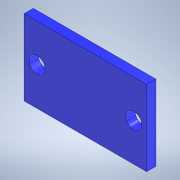
# Autodesk Inventor part: LogicLevelConverter
Saved by Autodesk Inventor 2021.2 (Build 252289000, 289)
## iProperties
Created: 2021-09-30
Part Number: LogicLevelConverter
Material: PET Plastic
Document SubType Name: Modeling
Designer: Roger
Density: 1.541 g/cm^3
Appearance: Blue - Wall Paint - Glossy
Author: Roger
Autodesk Inventor part; units mm, degrees
ref_plane "YZ Plane" through (0, 0, 0) normal (1, 0, 0) x (0, 1, 0)
ref_plane "XZ Plane" through (0, 0, 0) normal (0, 1, 0) x (-1, 0, 0)
ref_plane "XY Plane" through (0, 0, 0) normal (0, 0, 1) x (1, 0, 0)
sketch "Sketch1" plane through (0, 0, 0) normal (0, 0, 1) x (1, 0, 0)
  line L0 (-13.3, 8.2) -> (13.3, 8.2)
  line L1 (13.3, 8.2) -> (13.3, -8.2)
  line L2 (13.3, -8.2) -> (-13.3, -8.2)
  line L3 (-13.3, -8.2) -> (-13.3, 8.2)
  point P0 (0, 0)
  point P1 (-13.3, 0)
  point P2 (0, 8.2)
  dimension "d0" = 26.6
  dimension "d1" = 16.4
  constraints: 8 end point, 2 midpoint, 2 parallel, 1 horizontal, 1 horizontal alignment, 1 perpendicular, 1 vertical alignment
  measures "d0" distance of L0.start L0.end
  measures "d1" distance of L0.end L1.end
extrude "Extrusion1" add sketch "Sketch1" along normal blind 2
sketch "Sketch2" plane through (0, 0, 2) normal (0, 0, 1) x (1, 0, 0)
  circle A0 centre (-10.5, 0) radius 1.5
  circle A1 centre (10.5, 0) radius 1.5
  point P0 (0, 0)
  dimension "d4" = 3
  dimension "d5" = 21
  dimension "d6" = 10.5
  constraints: 2 centre point, 2 horizontal alignment, 1 equal radius
  measures "d4" diameter of A1
  measures "d5" distance of A1.centre A0.centre
  measures "d6" distance of A0.centre point (0, 0)
hole "Hole1" at (10.5, 0, 2) direction (0, 0, -1) diameter 3.5 end through all
pattern_linear "Rectangular Pattern1" count 2 spacing 21 along (-1, 0, 0) of "Hole1"
equation "\"d6\" = 0.5 * d5"
equation "\"d16\" = d5"
body "Solid1"
